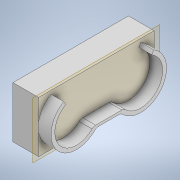
# Autodesk Inventor part: ultrasonic_fastening
Saved by Autodesk Inventor 2022 (Build 260153000, 153)
## iProperties
Created: 2022-02-09
Part Number: ultrasonic_fastening
Material: Generic
Document SubType Name: Modeling
Designer: Iñigo
Density: 1 g/cm^3
Appearance: Default
Author: Iñigo
Autodesk Inventor part; units mm, degrees
ref_plane "YZ Plane" through (0, 0, 0) normal (1, 0, 0) x (0, 1, 0)
ref_plane "XZ Plane" through (0, 0, 0) normal (0, 1, 0) x (-1, 0, 0)
ref_plane "XY Plane" through (0, 0, 0) normal (0, 0, 1) x (1, 0, 0)
sketch "Sketch1" plane through (0, 0, 0) normal (1, 0, 0) x (0, 1, 0)
  line L0 (10, 22.5) -> (-10, 22.5)
  line L1 (-10, 22.5) -> (-10, -22.5)
  line L2 (-10, -22.5) -> (10, -22.5)
  line L3 (10, -22.5) -> (10, 22.5)
  line L4 (10, 22.5) -> (-10, -22.5) construction
  line L5 (-10, 22.5) -> (10, -22.5) construction
  point P0 (0, 0)
  dimension "d0" = 20
  dimension "d1" = 45
  constraints: 12 end point, 2 midpoint, 2 parallel, 1 horizontal, 1 perpendicular
  measures "d0" distance of L2.end L1.end
  measures "d1" distance of L1.end L0.end
extrude "Extrusion1" add sketch "Sketch1" along normal blind 10
ref_plane "Work Plane1" through (10, 0, 0) normal (1, 0, 0) x (0, 0, -1)
sketch "Sketch2" plane through (10, 0, 0) normal (1, 0, 0) x (0, 0, -1)
  arc A0 (-16.9451, 7.3612) -> (-6.7165, -6.042) centre (-12.6951, 0) ccw
  arc A1 (-17.6951, 8.6603) -> (-5.5766, -7.0232) centre (-12.6951, 0) ccw
  line L0 (-0.1951, 8.5) -> (-0.1951, 4.1071)
  line L1 (-12.6951, 0) -> (-2.6951, 0) construction
  line L2 (-12.6951, 0) -> (-2.6951, 0) construction
  line L3 (-17.6951, 8.6603) -> (-16.9451, 7.3612)
  arc A2 (6.3262, -6.042) -> (16.5549, 7.3612) centre (12.3049, 0) ccw
  arc A3 (5.1863, -7.0232) -> (17.3049, 8.6603) centre (12.3049, 0) ccw
  line L4 (17.3049, 8.6603) -> (16.5549, 7.3612)
  line L5 (-5.3098, -5.4637) -> (4.9195, -5.4637)
  line L6 (-4.1528, -6.4279) -> (3.7626, -6.4279)
  arc A4 (-5.3098, -5.4637) -> (-6.7165, -6.042) centre (-5.3098, -7.4637) ccw
  arc A5 (6.3262, -6.042) -> (4.9195, -5.4637) centre (4.9195, -7.4637) ccw
  arc A6 (-4.1528, -6.4279) -> (-5.5766, -7.0232) centre (-4.1528, -8.4279) ccw
  arc A7 (5.1863, -7.0232) -> (3.7626, -6.4279) centre (3.7626, -8.4279) ccw
  point P0 (0, 0)
  point P1 (-5.0347, -6.4279)
  point P2 (4.6444, -6.4279)
  point P3 (5.7935, -5.4637)
  point P4 (4.6444, -6.4279)
  dimension "d6" = 20
  dimension "d10" = 12.5
  dimension "d16" = 2
  dimension "d17" = 2
  constraints: 18 point on circle, 14 end point, 8 centre point, 8 tangent, 5 symmetric about line, 3 point on line, 2 coincident, 2 equal radius, 2 horizontal, 1 vertical, 2 other
  measures "d6" diameter of A1
  measures "d10" distance from line of A0.centre L0
  measures "d16" radius of A4
  measures "d17" radius of A6
extrude "Extrusion2" add sketch "Sketch2" along normal blind 5
body "Solid1"
